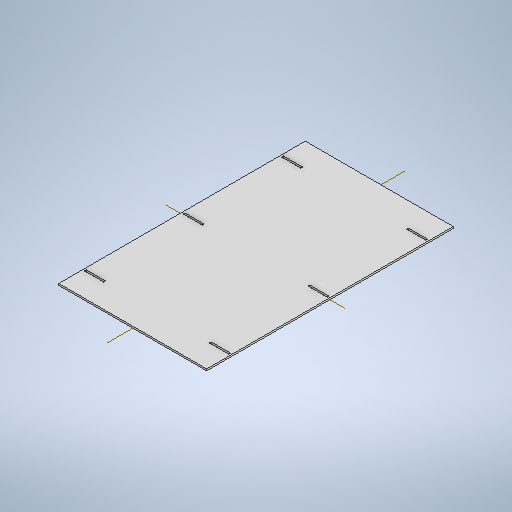
# Autodesk Inventor part: 부품1
Saved by Autodesk Inventor 2025 (Build 290162000, 162)
## iProperties
Created: 2024-04-04
Part Number: 부품1
Material: 일반
Document SubType Name: Modeling
Designer: gmsee
Density: 1 g/cm^3
Appearance: 기본값
Author: gmsee
Autodesk Inventor part; units mm, degrees
ref_plane "YZ Plane" through (0, 0, 0) normal (1, 0, 0) x (0, 1, 0)
ref_plane "XZ Plane" through (0, 0, 0) normal (0, 1, 0) x (-1, 0, 0)
ref_plane "XY Plane" through (0, 0, 0) normal (0, 0, 1) x (1, 0, 0)
sketch "스케치1" plane through (0, 0, 0) normal (0, 1, 0) x (-1, 0, 0)
  line L0 (150, 0) -> (150, -250)
  line L1 (150, -250) -> (0, -250)
  line L2 (210, 0) -> (-210, 0) projected
  line L3 (0, -350) -> (0, 350) projected
  line L4 (100, 0) -> (100, -250) construction
  line L5 (107.4, -198.15) -> (107.4, -201.85)
  line L6 (107.4, -201.85) -> (146.1, -201.85)
  line L7 (146.1, -198.15) -> (107.4, -198.15)
  line L8 (146.1, -201.85) -> (146.1, -198.15)
  line L9 (146.1, 0) -> (146.1, -1.85)
  line L10 (146.1, -1.85) -> (107.4, -1.85)
  line L11 (107.4, -1.85) -> (107.4, 0)
  line L12 (150, 0) -> (150, 250)
  line L13 (150, 250) -> (0, 250)
  line L14 (100, 0) -> (100, 250) construction
  line L15 (146.1, 198.15) -> (107.4, 198.15)
  line L16 (146.1, 201.85) -> (146.1, 198.15)
  line L17 (107.4, 201.85) -> (146.1, 201.85)
  line L18 (107.4, 198.15) -> (107.4, 201.85)
  line L19 (146.1, 0) -> (146.1, 1.85)
  line L20 (146.1, 1.85) -> (107.4, 1.85)
  line L21 (107.4, 1.85) -> (107.4, 0)
  line L22 (-150, 0) -> (-150, -250)
  line L23 (-150, -250) -> (0, -250)
  line L24 (-100, 0) -> (-100, -250) construction
  line L25 (-146.1, -198.15) -> (-107.4, -198.15)
  line L26 (-146.1, -201.85) -> (-146.1, -198.15)
  line L27 (-107.4, -201.85) -> (-146.1, -201.85)
  line L28 (-107.4, -198.15) -> (-107.4, -201.85)
  line L29 (-146.1, 0) -> (-146.1, -1.85)
  line L30 (-146.1, -1.85) -> (-107.4, -1.85)
  line L31 (-107.4, -1.85) -> (-107.4, 0)
  line L32 (-146.1, 1.85) -> (-107.4, 1.85)
  line L33 (-146.1, 0) -> (-146.1, 1.85)
  line L34 (-107.4, 1.85) -> (-107.4, 0)
  line L35 (-100, 0) -> (-100, 250) construction
  line L36 (-150, 0) -> (-150, 250)
  line L37 (-146.1, 198.15) -> (-107.4, 198.15)
  line L38 (-107.4, 198.15) -> (-107.4, 201.85)
  line L39 (-146.1, 201.85) -> (-146.1, 198.15)
  line L40 (-107.4, 201.85) -> (-146.1, 201.85)
  line L41 (-150, 250) -> (0, 250)
  point P0 (0, 0)
  dimension "d2" = 250
  dimension "d3" = 150
  dimension "d4" = 50
  dimension "d13" = 38.7
  dimension "d14" = 3.7
  dimension "d15" = 48.15
  dimension "d16" = 1.85
  dimension "d17" = 38.7
  dimension "d18" = 7.4
  dimension "d19" = 7.4
  constraints: 80 end point, 29 symmetric about line, 5 perpendicular, 4 point on line, 3 parallel, 1 horizontal, 1 vertical
  measures "d2" distance of L0.start L0.end
  measures "d3" distance of L0.end L1.end
  measures "d4" distance between parallel lines of L0 L4
  measures "d13" distance of L6.start L8.start
  measures "d14" distance of L7.end L6.start
  measures "d15" distance between parallel lines of L1 L6
  measures "d16" distance of L9.start L9.end
  measures "d17" distance of L9.end L10.end
  measures "d18" distance between parallel lines of L4 L11
  measures "d19" distance between parallel lines of L4 L5
extrude "돌출1" add sketch "스케치1" along normal blind 3.5 contours L0 L1 L3 L2 L11 L10 L9 | L2 L19 L20 L21 L3 L13 L12 | L23 L22 L2 L29 L30 L31 L3 | L3 L2 L34 L32 L33 L36 L41
